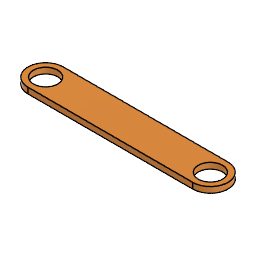
Bar (Autodesk Fusion 360 design; units mm, degrees)
part number: 2026-06-01-00-09-35-331
Autodesk Fusion 360 part; units mm, degrees
sketch "Sketch1" plane through (0, 0, 0) normal (0, 0, 1) x (1, 0, 0)
  circle A0 centre (14, 0) radius 2.05
  circle A1 centre (14, 0) radius 3
  circle A2 centre (-14, 0) radius 3
  circle A3 centre (-14, 0) radius 2.05
  line L0 (-14, 3) -> (14, 3)
  line L1 (-14, -3) -> (14, -3)
  line L2 (-14, 0) -> (14, 0) construction
  dimension "d1" = 4.1
  dimension "d2" = 6
  dimension "d3" = 28
  dimension "d4" = 6
  dimension "d5" = 4.1
  constraint concentric A0 A1
  constraint concentric A2 A3
  constraint coincident A2 L0.start
  constraint coincident A1 L0.end
  constraint tangent A1 L0
  constraint horizontal L0
  constraint coincident A2 L1.start
  constraint coincident A1 L1.end
  constraint tangent A1 L1
  constraint parallel L0 L1
  constraint coincident A2.centre A3.centre
  constraint coincident A0.centre A1.centre
  constraint midpoint origin L2
  measures "d1" diameter of A0
  measures "d2" diameter of A1
  measures "d3" distance of A0.centre A2.centre
  measures "d4" diameter of A2
  measures "d5" diameter of A3
extrude "Extrude1" add sketch "Sketch1" along normal blind 1
equation "d4 = d2"
equation "d5 = d1"
